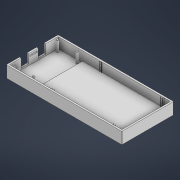
# Autodesk Inventor part: TOP
Saved by Autodesk Inventor 2022 (Build 260153000, 153)
## iProperties
Created: 2022-10-03
Part Number: TOP
Material: 常规
Document SubType Name: Modeling
Designer: 15628
Density: 1 g/cm^3
Appearance: 默认
Author: 15628
Autodesk Inventor part; units mm, degrees
ref_plane "YZ Plane" through (0, 0, 0) normal (1, 0, 0) x (0, 1, 0)
ref_plane "XZ Plane" through (0, 0, 0) normal (0, 1, 0) x (-1, 0, 0)
ref_plane "XY Plane" through (0, 0, 0) normal (0, 0, 1) x (1, 0, 0)
sketch "草图1" plane through (0, 0, 0) normal (0, 1, 0) x (-1, 0, 0)
  line L0 (0, 0) -> (0, -65)
  line L1 (0, -65) -> (145, -65)
  line L2 (145, -65) -> (145, 0)
  line L3 (145, 0) -> (0, 0)
  dimension "d0" = 65
  dimension "d2" = 145
  constraints: 8 end point, 2 perpendicular, 1 horizontal, 1 vertical
  measures "d0" distance of L0.start L0.end
  measures "d2" distance of L0.end L1.end
extrude "拉伸1" add sketch "草图1" along normal blind 15
sketch "草图2" plane through (0, 15, 0) normal (0, 1, 0) x (1, 0, 0)
  line L0 (-2, 2) -> (-2, 63)
  line L1 (-2, 63) -> (-143, 63)
  line L2 (-143, 63) -> (-143, 2)
  line L3 (-143, 2) -> (-2, 2)
  point P0 (0, 0)
  dimension "d5" = 61
  dimension "d6" = 141
  dimension "d7" = 61
  constraints: 8 end point, 2 perpendicular, 1 vertical
  measures "d5" distance of L0.start L0.end
  measures "d6" distance of L0.end L1.end
  measures "d7" distance of L1.end L2.end
extrude "拉伸2" cut sketch "草图2" against normal blind 13
sketch "草图3" plane through (0, 15, 0) normal (0, 1, 0) x (1, 0, 0)
  line L0 (-2, 2) -> (-143, 2) projected
  line L1 (-143, 2) -> (-143, 16.5)
  line L2 (-143, 2) -> (-143, 63) projected
  line L3 (-143, 16.5) -> (-143, 26)
  line L4 (-143, 26) -> (-143, 38)
  line L5 (-143, 38) -> (-143, 47.5)
  line L6 (-143, 47.5) -> (-145, 47.5)
  line L7 (-145, 65) -> (-145, 0) projected
  line L8 (-145, 47.5) -> (-145, 38)
  line L9 (-145, 38) -> (-143, 38)
  line L10 (-143, 26) -> (-145, 26)
  line L11 (-145, 26) -> (-145, 16.5)
  line L12 (-145, 16.5) -> (-143, 16.5)
  point P0 (0, 0)
  dimension "d10" = 14.5
  dimension "d11" = 9.5
  dimension "d12" = 12
  dimension "d13" = 9.5
  constraints: 20 end point, 7 point on line, 3 perpendicular, 2 parallel
  measures "d10" distance of L0.end L1.end
  measures "d11" distance of L1.end L3.end
  measures "d12" distance of L3.end L4.end
  measures "d13" distance of L4.end L5.end
extrude "拉伸3" cut sketch "草图3" against normal blind 11 contours L12 L7 L10 L2 | L9 L7 L6 L2
sketch "草图4" plane through (0, 2, 0) normal (0, 1, 0) x (1, 0, 0)
  line L0 (-143, 2) -> (-143, 63) projected
  line L1 (-143, 2) -> (-140.3334, 2)
  line L2 (-2, 2) -> (-143, 2) projected
  line L3 (-143, 2) -> (-140.3, 2)
  line L4 (-140.3, 2) -> (-140.3, 4.7)
  circle A0 centre (-140.3, 4.7) radius 1.5
  line L5 (-140.3, 4.7) -> (-140.3, 59.4)
  circle A1 centre (-140.3, 59.4) radius 1.5
  line L6 (-2, 63) -> (-2, 2) projected
  line L7 (-2, 2) -> (-12, 2)
  line L8 (-12, 2) -> (-12, 63)
  line L9 (-2, 2) -> (-89, 2)
  line L10 (-89, 2) -> (-89, 63)
  line L11 (-143, 63) -> (-2, 63) projected
  line L12 (-89, 63) -> (-90, 63)
  line L13 (-89, 63) -> (-88, 63)
  line L14 (-89, 63) -> (-90, 63)
  line L15 (-87, 63) -> (-86, 63)
  line L16 (-89, 63) -> (-90, 63)
  line L17 (-87, 63) -> (-86, 63)
  line L18 (-89, 63) -> (-88, 63)
  line L19 (-88, 63) -> (-88, 62)
  line L20 (-88, 62) -> (-87.5, 62)
  line L21 (-87.5, 62) -> (-87.5, 63)
  line L22 (-90, 63) -> (-90, 62)
  line L23 (-90, 62) -> (-90.5, 62)
  line L24 (-90.5, 62) -> (-90.5, 63)
  line L25 (-89, 2) -> (-88, 2)
  line L26 (-88, 2) -> (-88, 3)
  line L27 (-88, 3) -> (-87.5, 3)
  line L28 (-87.5, 3) -> (-87.5, 2)
  line L29 (-90, 3) -> (-90, 2)
  line L30 (-90, 3) -> (-90.5, 3)
  line L31 (-90.5, 3) -> (-90.5, 2)
  line L32 (-12, 63) -> (-11, 63)
  line L33 (-11, 63) -> (-11, 62)
  line L34 (-11, 62) -> (-10.5, 62)
  line L35 (-10.5, 62) -> (-10.5, 63)
  line L36 (-12, 63) -> (-13, 63)
  line L37 (-13, 63) -> (-13, 62)
  line L38 (-13, 62) -> (-13.5, 62)
  line L39 (-13.5, 62) -> (-13.5, 63)
  line L40 (-12, 2) -> (-11, 2)
  line L41 (-11, 2) -> (-11, 3)
  line L42 (-11, 3) -> (-10.5, 3)
  line L43 (-10.5, 3) -> (-10.5, 2)
  line L44 (-12, 2) -> (-13, 2)
  line L45 (-13, 2) -> (-13, 3)
  line L46 (-13, 3) -> (-13.5, 3)
  line L47 (-13.5, 3) -> (-13.5, 2)
  line L48 (-140.3, 59.4) -> (-115.535, 59.4)
  line L49 (-115.535, 59.4) -> (-115.535, 4.7)
  circle A2 centre (-115.535, 59.4) radius 1.5
  circle A3 centre (-115.535, 4.7) radius 1.5
  circle A4 centre (-115.535, 4.7) radius 1.4
  circle A5 centre (-115.535, 59.4) radius 1.4
  circle A6 centre (-140.3, 59.4) radius 1.4
  circle A7 centre (-140.3, 4.7) radius 1.4
  point P0 (0, 0)
  dimension "d19" = 2.7
  dimension "d20" = 2.7
  dimension "d21" = 3
  dimension "d22" = 54.7
  dimension "d23" = 3
  dimension "d28" = 10
  dimension "d29" = 87
  dimension "d44" = 1
  dimension "d45" = 1
  dimension "d46" = 0.5
  dimension "d47" = 0.5
  dimension "d48" = 1
  dimension "d49" = 1
  dimension "d50" = 0.5
  dimension "d51" = 0.5
  dimension "d52" = 1
  dimension "d53" = 1
  dimension "d54" = 0.5
  dimension "d55" = 1
  dimension "d56" = 0.5
  dimension "d57" = 1
  dimension "d58" = 1
  dimension "d59" = 0.5
  dimension "d60" = 1
  dimension "d61" = 1
  dimension "d65" = 24.765
  dimension "d66" = 3
  dimension "d67" = 3
  dimension "d71" = 2.8
  dimension "d72" = 2.8
  dimension "d73" = 2.8
  dimension "d74" = 2.8
  constraints: 92 end point, 34 point on line, 9 perpendicular, 8 centre point, 8 coincident, 4 vertical, 3 horizontal, 1 parallel, 10 other
  measures "d19" distance of L0.start L3.end
  measures "d20" distance of L3.end L4.end
  measures "d21" diameter of A0
  measures "d22" distance of L5.start L5.end
  measures "d23" diameter of A1
  measures "d28" distance of L2.start L7.end
  measures "d29" distance of L2.start L9.end
  measures "d44" distance of L16.start L13.end
  measures "d45" distance of L13.end L19.end
  measures "d46" distance of L19.end L20.end
  measures "d47" distance of L22.end L23.end
  measures "d48" distance of L9.end L25.end
  measures "d49" distance of L25.end L26.end
  measures "d50" distance of L26.end L27.end
  measures "d51" distance of L29.start L30.end
  measures "d52" distance of L8.end L32.end
  measures "d53" distance of L32.end L33.end
  measures "d54" distance of L33.end L34.end
  measures "d55" distance of L8.end L36.end
  measures "d56" distance of L37.end L38.end
  measures "d57" distance of L7.end L40.end
  measures "d58" distance of L40.end L41.end
  measures "d59" distance of L41.end L42.end
  measures "d60" distance of L7.end L44.end
  measures "d61" distance of L44.end L45.end
  measures "d65" distance of L48.start L48.end
  measures "d66" diameter of A2
  measures "d67" diameter of A3
  measures "d71" diameter of A4
  measures "d72" diameter of A5
  measures "d73" diameter of A6
  measures "d74" diameter of A7
extrude "拉伸4" add sketch "草图4" along normal blind 13 contours A4 | L11 L22 L23 L24 | L31 L30 L29 L2 | A7 L5 L4 | L4 L5 A7 | L11 L21 L20 L19 | L26 L27 L28 L2 | A6 L48 L5 | L5 L48 A6 | L47 L46 L45 L2 | A5 L49 L48 | L48 L49 A5 | L11 L37 L38 L39 | L41 L42 L43 L2 | L11 L35 L34 L33
sketch "草图5" plane through (0, 2, 0) normal (0, 1, 0) x (1, 0, 0)
  line L0 (-2, 63) -> (-2, 2) projected
  line L1 (-2, 63) -> (-112, 63)
  line L2 (-90, 63) -> (-88, 63) projected
  circle A0 centre (-115.535, 59.4) radius 1.5 projected
  line L3 (-115.535, 59.4) -> (-112.8683, 59.4)
  line L4 (-112, 63) -> (-112, 2)
  line L5 (-90.5, 2) -> (-143, 2) projected
  line L6 (-112, 63) -> (-2, 63)
  line L7 (-2, 63) -> (-2, 2) projected
  line L8 (-2, 63) -> (-2, 2)
  line L9 (-2, 2) -> (-112, 2)
  line L10 (-145, 0) -> (0, 0) projected
  dimension "d64" = 110
  dimension "d68" = 2.6667
  constraints: 12 end point, 2 collinear, 1 horizontal, 1 parallel, 1 perpendicular, 1 point on line, 1 vertical
  measures "d64" distance of L0.start L1.end
  measures "d68" distance of L3.start L3.end
extrude "拉伸5" add sketch "草图5" along normal blind 2 contours L0 L9 L5 L4 L1
sketch "草图6" plane through (-87.5, 15, -63) normal (0, 0, 1) x (1, 0, 0)
  line L0 (-2.5, 0) -> (-0.5, 0) projected
  line L1 (-0.5, 0) -> (-0.5, -4)
  line L2 (-0.5, -11) -> (-0.5, 0) projected
  line L3 (-0.5, -4) -> (-2.5, -4)
  line L4 (-2.5, 0) -> (-2.5, -11) projected
  line L5 (-2.5, 0) -> (-2.5, -4)
  line L6 (0, 0) -> (74, 0) projected
  line L7 (0, 0) -> (0, -4)
  line L8 (0, -11) -> (0, 0) projected
  line L9 (-1.1244, -4) -> (0, -4)
  line L10 (0, 0) -> (0, -4)
  line L11 (-0.5, -4) -> (-0.5, -6)
  line L12 (-0.5, -6) -> (-2.5, -6)
  line L13 (74.5, 0) -> (74.5, -6)
  line L14 (74.5, 0) -> (74.5, -11) projected
  line L15 (74.5, -6) -> (74.5, -4)
  line L16 (74.5, -4) -> (76.5, -4)
  line L17 (76.5, -11) -> (76.5, 0) projected
  line L18 (76.5, -4) -> (76.5, -6)
  line L19 (76.5, -6) -> (74.5, -6)
  point P0 (87.5, -15)
  dimension "d75" = 4
  dimension "d76" = 2
  dimension "d77" = 6
  dimension "d78" = 2
  constraints: 26 end point, 11 point on line, 6 perpendicular, 1 collinear
  measures "d75" distance of L0.end L1.end
  measures "d76" distance of L1.end L11.end
  measures "d77" distance of L13.start L13.end
  measures "d78" distance of L13.end L15.end
extrude "拉伸6" cut sketch "草图6" against normal blind 1 contours L3 L2 L12 L4 | L16 L17 L19 L13
sketch "草图7" plane through (-88, 15, -2) normal (0, 0, -1) x (-1, 0, 0)
  line L0 (0, 0) -> (0, -6)
  line L1 (0, 0) -> (0, -11) projected
  line L2 (0, -6) -> (0, -4)
  line L3 (0, -4) -> (2, -4)
  line L4 (2, -11) -> (2, 0) projected
  line L5 (0, -6) -> (2, -6)
  line L6 (2, -6) -> (2, -4)
  line L7 (-77, 0) -> (-77, -6)
  line L8 (-77, 0) -> (-77, -11) projected
  line L9 (-77, -6) -> (-75, -6)
  line L10 (-75, -11) -> (-75, 0) projected
  line L11 (-77, -6) -> (-77, -4)
  line L12 (-77, -4) -> (-75, -4)
  line L13 (-75, -4) -> (-75, -6)
  point P0 (-88, -15)
  point P1 (-75, -4)
  dimension "d81" = 6
  dimension "d82" = 2
  dimension "d83" = 6
  constraints: 20 end point, 9 point on line, 3 perpendicular, 1 horizontal
  measures "d81" distance of L0.start L0.end
  measures "d82" distance of L0.end L2.end
  measures "d83" distance of L7.start L7.end
extrude "拉伸7" cut sketch "草图7" against normal blind 1
chamfer "倒角1" distance 0.5 angle 45 33 edges at (-116.935, 15, -4.7) (-141.7, 15, -4.7) (-116.935, 15, -59.4) (-141.7, 15, -59.4) (-145, 0, -32.5) (-145, 7.5, -65) (-72.5, 0, -65) (-145, 7.5, 0) (-72.5, 0, 0) (0, 7.5, 0) (0, 0, -32.5) (0, 7.5, -65) (-50.5, 4, -63) (-101.25, 4, -63) (-89, 4, -63) (-12, 4, -63) (-6.25, 4, -63) (-2, 4, -32.5) (-6.25, 4, -2) (-12, 4, -2) (-50.5, 4, -2) (-89, 4, -2) (-101.25, 4, -2) (-90.5, 9.5, -2) (-13.5, 9.5, -2) (-87.5, 9.5, -2) (-10.5, 9.5, -2) (-87.5, 9.5, -63) (-10.5, 9.5, -63) (-90.5, 9.5, -63) (-13.5, 9.5, -63) (-2, 9.5, -63) (-2, 9.5, -2)
sketch "草图8" plane through (-143, 2, -2) normal (1, 0, 0) x (0, 0, -1)
  line L0 (24, 13) -> (24, 2) projected
  line L1 (24, 13) -> (24, 9)
  line L2 (24, 9) -> (36, 9)
  line L3 (36, 2) -> (36, 13) projected
  line L4 (36, 9) -> (36, 11)
  line L5 (36, 11) -> (24, 11)
  line L6 (24, 11) -> (25.5, 11)
  line L7 (25.5, 11) -> (25.5, 9)
  line L8 (36, 9) -> (34.5, 9)
  line L9 (34.5, 9) -> (34.5, 11)
  point P0 (-2, -2)
  dimension "d89" = 4
  dimension "d90" = 2
  dimension "d91" = 1.5
  dimension "d92" = 1.5
  constraints: 16 end point, 6 point on line, 3 perpendicular, 1 horizontal, 1 midpoint
  measures "d89" distance of L0.start L1.end
  measures "d90" distance of L2.end L4.end
  measures "d91" distance of L5.end L6.end
  measures "d92" distance of L2.end L8.end
extrude "拉伸8" cut sketch "草图8" against normal blind 1 contours L5 L9 L2 L7
